Autodesk Inventor part; units mm, degrees
(part 2 of 4)
  circle A543 centre (81.83, 22.3) radius 1.125
  circle A544 centre (8.17, 19.76) radius 1.125
  circle A545 centre (10.71, 19.76) radius 1.125
  circle A546 centre (13.25, 19.76) radius 1.125
  circle A547 centre (15.79, 19.76) radius 1.125
  circle A548 centre (18.33, 19.76) radius 1.125
  circle A549 centre (20.87, 19.76) radius 1.125
  circle A550 centre (23.41, 19.76) radius 1.125
  circle A551 centre (25.95, 19.76) radius 1.125
  circle A552 centre (28.49, 19.76) radius 1.125
  circle A553 centre (31.03, 19.76) radius 1.125
  circle A554 centre (33.57, 19.76) radius 1.125
  circle A555 centre (36.11, 19.76) radius 1.125
  circle A556 centre (38.65, 19.76) radius 1.125
  circle A557 centre (41.19, 19.76) radius 1.125
  circle A558 centre (43.73, 19.76) radius 1.125
  circle A559 centre (46.27, 19.76) radius 1.125
  circle A560 centre (48.81, 19.76) radius 1.125
  circle A561 centre (51.35, 19.76) radius 1.125
  circle A562 centre (53.89, 19.76) radius 1.125
  circle A563 centre (56.43, 19.76) radius 1.125
  circle A564 centre (58.97, 19.76) radius 1.125
  circle A565 centre (61.51, 19.76) radius 1.125
  circle A566 centre (64.05, 19.76) radius 1.125
  circle A567 centre (66.59, 19.76) radius 1.125
  circle A568 centre (69.13, 19.76) radius 1.125
  circle A569 centre (71.67, 19.76) radius 1.125
  circle A570 centre (74.21, 19.76) radius 1.125
  circle A571 centre (76.75, 19.76) radius 1.125
  circle A572 centre (79.29, 19.76) radius 1.125
  circle A573 centre (81.83, 19.76) radius 1.125
  circle A574 centre (8.17, 17.22) radius 1.125
  circle A575 centre (10.71, 17.22) radius 1.125
  circle A576 centre (13.25, 17.22) radius 1.125
  circle A577 centre (15.79, 17.22) radius 1.125
  circle A578 centre (18.33, 17.22) radius 1.125
  circle A579 centre (20.87, 17.22) radius 1.125
  circle A580 centre (23.41, 17.22) radius 1.125
  circle A581 centre (25.95, 17.22) radius 1.125
  circle A582 centre (28.49, 17.22) radius 1.125
  circle A583 centre (31.03, 17.22) radius 1.125
  circle A584 centre (33.57, 17.22) radius 1.125
  circle A585 centre (36.11, 17.22) radius 1.125
  circle A586 centre (38.65, 17.22) radius 1.125
  circle A587 centre (41.19, 17.22) radius 1.125
  circle A588 centre (43.73, 17.22) radius 1.125
  circle A589 centre (46.27, 17.22) radius 1.125
  circle A590 centre (48.81, 17.22) radius 1.125
  circle A591 centre (51.35, 17.22) radius 1.125
  circle A592 centre (53.89, 17.22) radius 1.125
  circle A593 centre (56.43, 17.22) radius 1.125
  circle A594 centre (58.97, 17.22) radius 1.125
  circle A595 centre (61.51, 17.22) radius 1.125
  circle A596 centre (64.05, 17.22) radius 1.125
  circle A597 centre (66.59, 17.22) radius 1.125
  circle A598 centre (69.13, 17.22) radius 1.125
  circle A599 centre (71.67, 17.22) radius 1.125
  circle A600 centre (74.21, 17.22) radius 1.125
  circle A601 centre (76.75, 17.22) radius 1.125
  circle A602 centre (79.29, 17.22) radius 1.125
  circle A603 centre (81.83, 17.22) radius 1.125
  circle A604 centre (8.17, 14.68) radius 1.125
  circle A605 centre (10.71, 14.68) radius 1.125
  circle A606 centre (13.25, 14.68) radius 1.125
  circle A607 centre (15.79, 14.68) radius 1.125
  circle A608 centre (18.33, 14.68) radius 1.125
  circle A609 centre (20.87, 14.68) radius 1.125
  circle A610 centre (23.41, 14.68) radius 1.125
  circle A611 centre (25.95, 14.68) radius 1.125
  circle A612 centre (28.49, 14.68) radius 1.125
  circle A613 centre (31.03, 14.68) radius 1.125
  circle A614 centre (33.57, 14.68) radius 1.125
  circle A615 centre (36.11, 14.68) radius 1.125
  circle A616 centre (38.65, 14.68) radius 1.125
  circle A617 centre (41.19, 14.68) radius 1.125
  circle A618 centre (43.73, 14.68) radius 1.125
  circle A619 centre (46.27, 14.68) radius 1.125
  circle A620 centre (48.81, 14.68) radius 1.125
  circle A621 centre (51.35, 14.68) radius 1.125
  circle A622 centre (53.89, 14.68) radius 1.125
  circle A623 centre (56.43, 14.68) radius 1.125
  circle A624 centre (58.97, 14.68) radius 1.125
  circle A625 centre (61.51, 14.68) radius 1.125
  circle A626 centre (64.05, 14.68) radius 1.125
  circle A627 centre (66.59, 14.68) radius 1.125
  circle A628 centre (69.13, 14.68) radius 1.125
  circle A629 centre (71.67, 14.68) radius 1.125
  circle A630 centre (74.21, 14.68) radius 1.125
  circle A631 centre (76.75, 14.68) radius 1.125
  circle A632 centre (79.29, 14.68) radius 1.125
  circle A633 centre (81.83, 14.68) radius 1.125
  circle A634 centre (8.17, 12.14) radius 1.125
  circle A635 centre (10.71, 12.14) radius 1.125
  circle A636 centre (13.25, 12.14) radius 1.125
  circle A637 centre (15.79, 12.14) radius 1.125
  circle A638 centre (18.33, 12.14) radius 1.125
  circle A639 centre (20.87, 12.14) radius 1.125
  circle A640 centre (23.41, 12.14) radius 1.125
  circle A641 centre (25.95, 12.14) radius 1.125
  circle A642 centre (28.49, 12.14) radius 1.125
  circle A643 centre (31.03, 12.14) radius 1.125
  circle A644 centre (33.57, 12.14) radius 1.125
  circle A645 centre (36.11, 12.14) radius 1.125
  circle A646 centre (38.65, 12.14) radius 1.125
  circle A647 centre (41.19, 12.14) radius 1.125
  circle A648 centre (43.73, 12.14) radius 1.125
  circle A649 centre (46.27, 12.14) radius 1.125
  circle A650 centre (48.81, 12.14) radius 1.125
  circle A651 centre (51.35, 12.14) radius 1.125
  circle A652 centre (53.89, 12.14) radius 1.125
  circle A653 centre (56.43, 12.14) radius 1.125
  circle A654 centre (58.97, 12.14) radius 1.125
  circle A655 centre (61.51, 12.14) radius 1.125
  circle A656 centre (64.05, 12.14) radius 1.125
  circle A657 centre (66.59, 12.14) radius 1.125
  circle A658 centre (69.13, 12.14) radius 1.125
  circle A659 centre (71.67, 12.14) radius 1.125
  circle A660 centre (74.21, 12.14) radius 1.125
  circle A661 centre (76.75, 12.14) radius 1.125
  circle A662 centre (79.29, 12.14) radius 1.125
  circle A663 centre (81.83, 12.14) radius 1.125
  circle A664 centre (8.17, 9.6) radius 1.125
  circle A665 centre (10.71, 9.6) radius 1.125
  circle A666 centre (13.25, 9.6) radius 1.125
  circle A667 centre (15.79, 9.6) radius 1.125
  circle A668 centre (18.33, 9.6) radius 1.125
  circle A669 centre (20.87, 9.6) radius 1.125
  circle A670 centre (23.41, 9.6) radius 1.125
  circle A671 centre (25.95, 9.6) radius 1.125
  circle A672 centre (28.49, 9.6) radius 1.125
  circle A673 centre (31.03, 9.6) radius 1.125
  circle A674 centre (33.57, 9.6) radius 1.125
  circle A675 centre (36.11, 9.6) radius 1.125
  circle A676 centre (38.65, 9.6) radius 1.125
  circle A677 centre (41.19, 9.6) radius 1.125
  circle A678 centre (43.73, 9.6) radius 1.125
  circle A679 centre (46.27, 9.6) radius 1.125
  circle A680 centre (48.81, 9.6) radius 1.125
  circle A681 centre (51.35, 9.6) radius 1.125
  circle A682 centre (53.89, 9.6) radius 1.125
  circle A683 centre (56.43, 9.6) radius 1.125
  circle A684 centre (58.97, 9.6) radius 1.125
  circle A685 centre (61.51, 9.6) radius 1.125
  circle A686 centre (64.05, 9.6) radius 1.125
  circle A687 centre (66.59, 9.6) radius 1.125
  circle A688 centre (69.13, 9.6) radius 1.125
  circle A689 centre (71.67, 9.6) radius 1.125
  circle A690 centre (74.21, 9.6) radius 1.125
  circle A691 centre (76.75, 9.6) radius 1.125
  circle A692 centre (79.29, 9.6) radius 1.125
  circle A693 centre (81.83, 9.6) radius 1.125
  circle A694 centre (8.17, 7.06) radius 1.125
  circle A695 centre (10.71, 7.06) radius 1.125
  circle A696 centre (13.25, 7.06) radius 1.125
  circle A697 centre (15.79, 7.06) radius 1.125
  circle A698 centre (18.33, 7.06) radius 1.125
  circle A699 centre (20.87, 7.06) radius 1.125
  circle A700 centre (23.41, 7.06) radius 1.125
  circle A701 centre (25.95, 7.06) radius 1.125
  circle A702 centre (28.49, 7.06) radius 1.125
  circle A703 centre (31.03, 7.06) radius 1.125
  circle A704 centre (33.57, 7.06) radius 1.125
  circle A705 centre (36.11, 7.06) radius 1.125
  circle A706 centre (38.65, 7.06) radius 1.125
  circle A707 centre (41.19, 7.06) radius 1.125
  circle A708 centre (43.73, 7.06) radius 1.125
  circle A709 centre (46.27, 7.06) radius 1.125
  circle A710 centre (48.81, 7.06) radius 1.125
  circle A711 centre (51.35, 7.06) radius 1.125
  circle A712 centre (53.89, 7.06) radius 1.125
  circle A713 centre (56.43, 7.06) radius 1.125
  circle A714 centre (58.97, 7.06) radius 1.125
  circle A715 centre (61.51, 7.06) radius 1.125
  circle A716 centre (64.05, 7.06) radius 1.125
  circle A717 centre (66.59, 7.06) radius 1.125
  circle A718 centre (69.13, 7.06) radius 1.125
  circle A719 centre (71.67, 7.06) radius 1.125
  circle A720 centre (74.21, 7.06) radius 1.125
  circle A721 centre (76.75, 7.06) radius 1.125
  circle A722 centre (79.29, 7.06) radius 1.125
  circle A723 centre (81.83, 7.06) radius 1.125
  circle A724 centre (8.17, 4.52) radius 1.125
  circle A725 centre (10.71, 4.52) radius 1.125
  circle A726 centre (13.25, 4.52) radius 1.125
  circle A727 centre (15.79, 4.52) radius 1.125
  circle A728 centre (18.33, 4.52) radius 1.125
  circle A729 centre (20.87, 4.52) radius 1.125
  circle A730 centre (23.41, 4.52) radius 1.125
  circle A731 centre (25.95, 4.52) radius 1.125
  circle A732 centre (28.49, 4.52) radius 1.125
  circle A733 centre (31.03, 4.52) radius 1.125
  circle A734 centre (33.57, 4.52) radius 1.125
  circle A735 centre (36.11, 4.52) radius 1.125
  circle A736 centre (38.65, 4.52) radius 1.125
  circle A737 centre (41.19, 4.52) radius 1.125
  circle A738 centre (43.73, 4.52) radius 1.125
  circle A739 centre (46.27, 4.52) radius 1.125
  circle A740 centre (48.81, 4.52) radius 1.125
  circle A741 centre (51.35, 4.52) radius 1.125
  circle A742 centre (53.89, 4.52) radius 1.125
  circle A743 centre (56.43, 4.52) radius 1.125
  circle A744 centre (58.97, 4.52) radius 1.125
  circle A745 centre (61.51, 4.52) radius 1.125
  circle A746 centre (64.05, 4.52) radius 1.125
  circle A747 centre (66.59, 4.52) radius 1.125
  circle A748 centre (69.13, 4.52) radius 1.125
  circle A749 centre (71.67, 4.52) radius 1.125
  circle A750 centre (74.21, 4.52) radius 1.125
  circle A751 centre (76.75, 4.52) radius 1.125
  circle A752 centre (79.29, 4.52) radius 1.125
  circle A753 centre (81.83, 4.52) radius 1.125
  line L4 (0, 70) -> (0, 0) construction
  line L5 (0, 35) -> (90, 35) construction
  line L6 (45, 70) -> (45, 0) construction
  line L7 (0, 0) -> (90, 0) construction
  line L8 (43.73, 65.48) -> (46.27, 65.48) construction
  point P0 (45, 65.48)
  dimension "d9" = 2.25
  dimension "d12" = 2.54
  dimension "d15" = 2.54
  constraints: 750 centre point, 6 end point, 5 midpoint, 2 horizontal, 2 point on line, 1 vertical, 1498 other
  measures "d9" diameter of A0
  measures "d12" distance of A0.centre A5.centre
  measures "d15" distance of A0.centre A34.centre
extrude "PCB_Pads" add sketch "Sketch3" along normal blind 0.05
sketch "Sketch6" plane through (0, 0, 0) normal (0, -1, 0) x (1, 0, 0)
  arc A0 (2.6, -13.65) -> (2.6, -16.35) centre (2.6, -15) ccw construction
  line L0 (2.6, -16.35) -> (4.9, -16.35) construction
  arc A1 (4.9, -16.35) -> (4.9, -13.65) centre (4.9, -15) ccw construction
  line L1 (4.9, -13.65) -> (2.6, -13.65) construction
  arc A2 (2.6, -21.65) -> (2.6, -24.35) centre (2.6, -23) ccw construction
  line L2 (2.6, -24.35) -> (4.9, -24.35) construction
  arc A3 (4.9, -24.35) -> (4.9, -21.65) centre (4.9, -23) ccw construction
  line L3 (4.9, -21.65) -> (2.6, -21.65) construction
  arc A4 (2.6, -49.65) -> (2.6, -52.35) centre (2.6, -51) ccw construction
  line L4 (2.6, -52.35) -> (4.9, -52.35) construction
  arc A5 (4.9, -52.35) -> (4.9, -49.65) centre (4.9, -51) ccw construction
  line L5 (4.9, -49.65) -> (2.6, -49.65) construction
  arc A6 (2.6, -37.65) -> (2.6, -40.35) centre (2.6, -39) ccw construction
  line L6 (2.6, -40.35) -> (4.9, -40.35) construction
  arc A7 (4.9, -40.35) -> (4.9, -37.65) centre (4.9, -39) ccw construction
  line L7 (4.9, -37.65) -> (2.6, -37.65) construction
  arc A8 (2.6, -57.65) -> (2.6, -60.35) centre (2.6, -59) ccw construction
  line L8 (2.6, -60.35) -> (4.9, -60.35) construction
  arc A9 (4.9, -60.35) -> (4.9, -57.65) centre (4.9, -59) ccw construction
  line L9 (4.9, -57.65) -> (2.6, -57.65) construction
  arc A10 (2.6, -41.65) -> (2.6, -44.35) centre (2.6, -43) ccw construction
  line L10 (2.6, -44.35) -> (4.9, -44.35) construction
  arc A11 (4.9, -44.35) -> (4.9, -41.65) centre (4.9, -43) ccw construction
  line L11 (4.9, -41.65) -> (2.6, -41.65) construction
  arc A12 (85.1, -9.65) -> (85.1, -12.35) centre (85.1, -11) ccw construction
  line L12 (85.1, -12.35) -> (87.4, -12.35) construction
  arc A13 (87.4, -12.35) -> (87.4, -9.65) centre (87.4, -11) ccw construction
  line L13 (87.4, -9.65) -> (85.1, -9.65) construction
  arc A14 (85.1, -17.65) -> (85.1, -20.35) centre (85.1, -19) ccw construction
  line L14 (85.1, -20.35) -> (87.4, -20.35) construction
  arc A15 (87.4, -20.35) -> (87.4, -17.65) centre (87.4, -19) ccw construction
  line L15 (87.4, -17.65) -> (85.1, -17.65) construction
  arc A16 (85.1, -25.65) -> (85.1, -28.35) centre (85.1, -27) ccw construction
  line L16 (85.1, -28.35) -> (87.4, -28.35) construction
  arc A17 (87.4, -28.35) -> (87.4, -25.65) centre (87.4, -27) ccw construction
  line L17 (87.4, -25.65) -> (85.1, -25.65) construction
  arc A18 (85.1, -57.65) -> (85.1, -60.35) centre (85.1, -59) ccw construction
  line L18 (85.1, -60.35) -> (87.4, -60.35) construction
  arc A19 (87.4, -60.35) -> (87.4, -57.65) centre (87.4, -59) ccw construction
  line L19 (87.4, -57.65) -> (85.1, -57.65) construction
  arc A20 (85.1, -49.65) -> (85.1, -52.35) centre (85.1, -51) ccw construction
  line L20 (85.1, -52.35) -> (87.4, -52.35) construction
  arc A21 (87.4, -52.35) -> (87.4, -49.65) centre (87.4, -51) ccw construction
  line L21 (87.4, -49.65) -> (85.1, -49.65) construction
  arc A22 (85.1, -41.65) -> (85.1, -44.35) centre (85.1, -43) ccw construction
  line L22 (85.1, -44.35) -> (87.4, -44.35) construction
  arc A23 (87.4, -44.35) -> (87.4, -41.65) centre (87.4, -43) ccw construction
  line L23 (87.4, -41.65) -> (85.1, -41.65) construction
  arc A24 (87.4, -36.35) -> (87.4, -33.65) centre (87.4, -35) ccw construction
  line L24 (87.4, -33.65) -> (85.1, -33.65) construction
  arc A25 (85.1, -33.65) -> (85.1, -36.35) centre (85.1, -35) ccw construction
  line L25 (85.1, -36.35) -> (87.4, -36.35) construction
  arc A26 (85.1, -37.65) -> (85.1, -40.35) centre (85.1, -39) ccw construction
  line L26 (85.1, -40.35) -> (87.4, -40.35) construction
  arc A27 (87.4, -40.35) -> (87.4, -37.65) centre (87.4, -39) ccw construction
  line L27 (87.4, -37.65) -> (85.1, -37.65) construction
  arc A28 (85.1, -45.65) -> (85.1, -48.35) centre (85.1, -47) ccw construction
  line L28 (85.1, -48.35) -> (87.4, -48.35) construction
  arc A29 (87.4, -48.35) -> (87.4, -45.65) centre (87.4, -47) ccw construction
  line L29 (87.4, -45.65) -> (85.1, -45.65) construction
  arc A30 (85.1, -53.65) -> (85.1, -56.35) centre (85.1, -55) ccw construction
  line L30 (85.1, -56.35) -> (87.4, -56.35) construction
  arc A31 (87.4, -56.35) -> (87.4, -53.65) centre (87.4, -55) ccw construction
  line L31 (87.4, -53.65) -> (85.1, -53.65) construction
  arc A32 (85.1, -29.65) -> (85.1, -32.35) centre (85.1, -31) ccw construction
  line L32 (85.1, -32.35) -> (87.4, -32.35) construction
  arc A33 (87.4, -32.35) -> (87.4, -29.65) centre (87.4, -31) ccw construction
  line L33 (87.4, -29.65) -> (85.1, -29.65) construction
  arc A34 (85.1, -21.65) -> (85.1, -24.35) centre (85.1, -23) ccw construction
  line L34 (85.1, -24.35) -> (87.4, -24.35) construction
  arc A35 (87.4, -24.35) -> (87.4, -21.65) centre (87.4, -23) ccw construction
  line L35 (87.4, -21.65) -> (85.1, -21.65) construction
  arc A36 (85.1, -13.65) -> (85.1, -16.35) centre (85.1, -15) ccw construction
  line L36 (85.1, -16.35) -> (87.4, -16.35) construction
  arc A37 (87.4, -16.35) -> (87.4, -13.65) centre (87.4, -15) ccw construction
  line L37 (87.4, -13.65) -> (85.1, -13.65) construction
  arc A38 (4.9, -36.35) -> (4.9, -33.65) centre (4.9, -35) ccw construction
  line L38 (4.9, -33.65) -> (2.6, -33.65) construction
  arc A39 (2.6, -33.65) -> (2.6, -36.35) centre (2.6, -35) ccw construction
  line L39 (2.6, -36.35) -> (4.9, -36.35) construction
  arc A40 (2.6, -53.65) -> (2.6, -56.35) centre (2.6, -55) ccw construction
  line L40 (2.6, -56.35) -> (4.9, -56.35) construction
  arc A41 (4.9, -56.35) -> (4.9, -53.65) centre (4.9, -55) ccw construction
  line L41 (4.9, -53.65) -> (2.6, -53.65) construction
  arc A42 (2.6, -29.65) -> (2.6, -32.35) centre (2.6, -31) ccw construction
  line L42 (2.6, -32.35) -> (4.9, -32.35) construction
  arc A43 (4.9, -32.35) -> (4.9, -29.65) centre (4.9, -31) ccw construction
  line L43 (4.9, -29.65) -> (2.6, -29.65) construction
  arc A44 (2.6, -45.65) -> (2.6, -48.35) centre (2.6, -47) ccw construction
  line L44 (2.6, -48.35) -> (4.9, -48.35) construction
  arc A45 (4.9, -48.35) -> (4.9, -45.65) centre (4.9, -47) ccw construction
  line L45 (4.9, -45.65) -> (2.6, -45.65) construction
  arc A46 (2.6, -25.65) -> (2.6, -28.35) centre (2.6, -27) ccw construction
  line L46 (2.6, -28.35) -> (4.9, -28.35) construction
  arc A47 (4.9, -28.35) -> (4.9, -25.65) centre (4.9, -27) ccw construction
  line L47 (4.9, -25.65) -> (2.6, -25.65) construction
  arc A48 (4.9, -20.35) -> (4.9, -17.65) centre (4.9, -19) ccw construction
  line L48 (4.9, -17.65) -> (2.6, -17.65) construction
  arc A49 (2.6, -17.65) -> (2.6, -20.35) centre (2.6, -19) ccw construction
  line L49 (2.6, -20.35) -> (4.9, -20.35) construction
  arc A50 (2.6, -9.65) -> (2.6, -12.35) centre (2.6, -11) ccw construction
  line L50 (2.6, -12.35) -> (4.9, -12.35) construction
  arc A51 (4.9, -12.35) -> (4.9, -9.65) centre (4.9, -11) ccw construction
  line L51 (4.9, -9.65) -> (2.6, -9.65) construction
  circle A52 centre (79.29, -4.52) radius 1.125 construction
  circle A53 centre (74.21, -4.52) radius 1.125 construction
  circle A54 centre (69.13, -4.52) radius 1.125 construction
  circle A55 centre (64.05, -4.52) radius 1.125 construction
  circle A56 centre (58.97, -4.52) radius 1.125 construction
  circle A57 centre (53.89, -4.52) radius 1.125 construction
  circle A58 centre (48.81, -4.52) radius 1.125 construction
  circle A59 centre (43.73, -4.52) radius 1.125 construction
  circle A60 centre (38.65, -4.52) radius 1.125 construction
  circle A61 centre (33.57, -4.52) radius 1.125 construction
  circle A62 centre (28.49, -4.52) radius 1.125 construction
  circle A63 centre (23.41, -4.52) radius 1.125 construction
  circle A64 centre (18.33, -4.52) radius 1.125 construction
  circle A65 centre (13.25, -4.52) radius 1.125 construction
  circle A66 centre (8.17, -4.52) radius 1.125 construction
  circle A67 centre (79.29, -7.06) radius 1.125 construction
  circle A68 centre (74.21, -7.06) radius 1.125 construction
  circle A69 centre (69.13, -7.06) radius 1.125 construction
  circle A70 centre (64.05, -7.06) radius 1.125 construction
  circle A71 centre (58.97, -7.06) radius 1.125 construction
  circle A72 centre (53.89, -7.06) radius 1.125 construction
  circle A73 centre (48.81, -7.06) radius 1.125 construction
  circle A74 centre (43.73, -7.06) radius 1.125 construction
  circle A75 centre (38.65, -7.06) radius 1.125 construction
  circle A76 centre (33.57, -7.06) radius 1.125 construction
  circle A77 centre (28.49, -7.06) radius 1.125 construction
  circle A78 centre (23.41, -7.06) radius 1.125 construction
  circle A79 centre (18.33, -7.06) radius 1.125 construction
  circle A80 centre (13.25, -7.06) radius 1.125 construction
  circle A81 centre (8.17, -7.06) radius 1.125 construction
  circle A82 centre (79.29, -9.6) radius 1.125 construction
  circle A83 centre (74.21, -9.6) radius 1.125 construction
  circle A84 centre (69.13, -9.6) radius 1.125 construction
  circle A85 centre (64.05, -9.6) radius 1.125 construction
  circle A86 centre (58.97, -9.6) radius 1.125 construction
  circle A87 centre (53.89, -9.6) radius 1.125 construction
  circle A88 centre (48.81, -9.6) radius 1.125 construction
  circle A89 centre (43.73, -9.6) radius 1.125 construction
  circle A90 centre (38.65, -9.6) radius 1.125 construction
  circle A91 centre (33.57, -9.6) radius 1.125 construction
  circle A92 centre (28.49, -9.6) radius 1.125 construction
  circle A93 centre (23.41, -9.6) radius 1.125 construction
  circle A94 centre (18.33, -9.6) radius 1.125 construction
  circle A95 centre (13.25, -9.6) radius 1.125 construction
  circle A96 centre (8.17, -9.6) radius 1.125 construction
  circle A97 centre (79.29, -12.14) radius 1.125 construction
  circle A98 centre (74.21, -12.14) radius 1.125 construction
  circle A99 centre (69.13, -12.14) radius 1.125 construction
  circle A100 centre (64.05, -12.14) radius 1.125 construction
  circle A101 centre (58.97, -12.14) radius 1.125 construction
  circle A102 centre (53.89, -12.14) radius 1.125 construction
  circle A103 centre (48.81, -12.14) radius 1.125 construction
  circle A104 centre (43.73, -12.14) radius 1.125 construction
  circle A105 centre (38.65, -12.14) radius 1.125 construction
  circle A106 centre (33.57, -12.14) radius 1.125 construction
  circle A107 centre (28.49, -12.14) radius 1.125 construction
  circle A108 centre (23.41, -12.14) radius 1.125 construction
  circle A109 centre (18.33, -12.14) radius 1.125 construction
  circle A110 centre (13.25, -12.14) radius 1.125 construction
  circle A111 centre (8.17, -12.14) radius 1.125 construction
  circle A112 centre (79.29, -14.68) radius 1.125 construction
  circle A113 centre (74.21, -14.68) radius 1.125 construction
  circle A114 centre (69.13, -14.68) radius 1.125 construction
  circle A115 centre (64.05, -14.68) radius 1.125 construction
  circle A116 centre (58.97, -14.68) radius 1.125 construction
  circle A117 centre (53.89, -14.68) radius 1.125 construction
  circle A118 centre (48.81, -14.68) radius 1.125 construction
  circle A119 centre (43.73, -14.68) radius 1.125 construction
  circle A120 centre (38.65, -14.68) radius 1.125 construction
  circle A121 centre (33.57, -14.68) radius 1.125 construction
  circle A122 centre (28.49, -14.68) radius 1.125 construction
  circle A123 centre (23.41, -14.68) radius 1.125 construction
  circle A124 centre (18.33, -14.68) radius 1.125 construction
  circle A125 centre (13.25, -14.68) radius 1.125 construction
  circle A126 centre (8.17, -14.68) radius 1.125 construction
  circle A127 centre (79.29, -17.22) radius 1.125 construction
  circle A128 centre (74.21, -17.22) radius 1.125 construction
  circle A129 centre (69.13, -17.22) radius 1.125 construction
  circle A130 centre (64.05, -17.22) radius 1.125 construction
  circle A131 centre (58.97, -17.22) radius 1.125 construction
  circle A132 centre (53.89, -17.22) radius 1.125 construction
  circle A133 centre (48.81, -17.22) radius 1.125 construction
  circle A134 centre (43.73, -17.22) radius 1.125 construction
  circle A135 centre (38.65, -17.22) radius 1.125 construction
  circle A136 centre (33.57, -17.22) radius 1.125 construction
  circle A137 centre (28.49, -17.22) radius 1.125 construction
  circle A138 centre (23.41, -17.22) radius 1.125 construction
  circle A139 centre (18.33, -17.22) radius 1.125 construction
  circle A140 centre (13.25, -17.22) radius 1.125 construction
  circle A141 centre (8.17, -17.22) radius 1.125 construction
  circle A142 centre (79.29, -19.76) radius 1.125 construction
  circle A143 centre (74.21, -19.76) radius 1.125 construction
  circle A144 centre (69.13, -19.76) radius 1.125 construction
  circle A145 centre (64.05, -19.76) radius 1.125 construction
  circle A146 centre (58.97, -19.76) radius 1.125 construction
  circle A147 centre (53.89, -19.76) radius 1.125 construction
  circle A148 centre (48.81, -19.76) radius 1.125 construction
  circle A149 centre (43.73, -19.76) radius 1.125 construction
  circle A150 centre (38.65, -19.76) radius 1.125 construction
  circle A151 centre (33.57, -19.76) radius 1.125 construction
  circle A152 centre (28.49, -19.76) radius 1.125 construction
  circle A153 centre (23.41, -19.76) radius 1.125 construction
  circle A154 centre (18.33, -19.76) radius 1.125 construction
  circle A155 centre (13.25, -19.76) radius 1.125 construction
  circle A156 centre (8.17, -19.76) radius 1.125 construction
  circle A157 centre (79.29, -22.3) radius 1.125 construction
  circle A158 centre (74.21, -22.3) radius 1.125 construction
  circle A159 centre (69.13, -22.3) radius 1.125 construction
  circle A160 centre (64.05, -22.3) radius 1.125 construction
  circle A161 centre (58.97, -22.3) radius 1.125 construction
  circle A162 centre (53.89, -22.3) radius 1.125 construction
  circle A163 centre (48.81, -22.3) radius 1.125 construction
  circle A164 centre (43.73, -22.3) radius 1.125 construction
  circle A165 centre (38.65, -22.3) radius 1.125 construction
  circle A166 centre (33.57, -22.3) radius 1.125 construction
  circle A167 centre (28.49, -22.3) radius 1.125 construction
  circle A168 centre (23.41, -22.3) radius 1.125 construction
  circle A169 centre (18.33, -22.3) radius 1.125 construction
  circle A170 centre (13.25, -22.3) radius 1.125 construction
  circle A171 centre (8.17, -22.3) radius 1.125 construction
  circle A172 centre (79.29, -24.84) radius 1.125 construction
  circle A173 centre (74.21, -24.84) radius 1.125 construction
  circle A174 centre (69.13, -24.84) radius 1.125 construction
  circle A175 centre (64.05, -24.84) radius 1.125 construction
  circle A176 centre (58.97, -24.84) radius 1.125 construction
  circle A177 centre (53.89, -24.84) radius 1.125 construction
  circle A178 centre (48.81, -24.84) radius 1.125 construction
  circle A179 centre (43.73, -24.84) radius 1.125 construction
  circle A180 centre (38.65, -24.84) radius 1.125 construction
  circle A181 centre (33.57, -24.84) radius 1.125 construction
  circle A182 centre (28.49, -24.84) radius 1.125 construction
  circle A183 centre (23.41, -24.84) radius 1.125 construction
  circle A184 centre (18.33, -24.84) radius 1.125 construction
  circle A185 centre (13.25, -24.84) radius 1.125 construction
  circle A186 centre (8.17, -24.84) radius 1.125 construction
  circle A187 centre (79.29, -27.38) radius 1.125 construction
  circle A188 centre (74.21, -27.38) radius 1.125 construction
  circle A189 centre (69.13, -27.38) radius 1.125 construction
  circle A190 centre (64.05, -27.38) radius 1.125 construction
  circle A191 centre (58.97, -27.38) radius 1.125 construction
  circle A192 centre (53.89, -27.38) radius 1.125 construction
  circle A193 centre (48.81, -27.38) radius 1.125 construction
  circle A194 centre (43.73, -27.38) radius 1.125 construction
  circle A195 centre (38.65, -27.38) radius 1.125 construction
  circle A196 centre (33.57, -27.38) radius 1.125 construction
  circle A197 centre (28.49, -27.38) radius 1.125 construction
  circle A198 centre (23.41, -27.38) radius 1.125 construction
  circle A199 centre (18.33, -27.38) radius 1.125 construction
  circle A200 centre (13.25, -27.38) radius 1.125 construction
  circle A201 centre (8.17, -27.38) radius 1.125 construction
  circle A202 centre (79.29, -29.92) radius 1.125 construction
  circle A203 centre (74.21, -29.92) radius 1.125 construction
  circle A204 centre (69.13, -29.92) radius 1.125 construction
  circle A205 centre (64.05, -29.92) radius 1.125 construction
  circle A206 centre (58.97, -29.92) radius 1.125 construction
  circle A207 centre (53.89, -29.92) radius 1.125 construction
  circle A208 centre (48.81, -29.92) radius 1.125 construction
  circle A209 centre (43.73, -29.92) radius 1.125 construction
  circle A210 centre (38.65, -29.92) radius 1.125 construction
  circle A211 centre (33.57, -29.92) radius 1.125 construction
  circle A212 centre (28.49, -29.92) radius 1.125 construction
  circle A213 centre (23.41, -29.92) radius 1.125 construction
  circle A214 centre (18.33, -29.92) radius 1.125 construction
  circle A215 centre (13.25, -29.92) radius 1.125 construction
  circle A216 centre (8.17, -29.92) radius 1.125 construction
  circle A217 centre (79.29, -32.46) radius 1.125 construction
  circle A218 centre (74.21, -32.46) radius 1.125 construction
  circle A219 centre (69.13, -32.46) radius 1.125 construction
  circle A220 centre (64.05, -32.46) radius 1.125 construction
  circle A221 centre (58.97, -32.46) radius 1.125 construction
  circle A222 centre (53.89, -32.46) radius 1.125 construction
  circle A223 centre (48.81, -32.46) radius 1.125 construction
  circle A224 centre (43.73, -32.46) radius 1.125 construction
  circle A225 centre (38.65, -32.46) radius 1.125 construction
  circle A226 centre (33.57, -32.46) radius 1.125 construction
  circle A227 centre (28.49, -32.46) radius 1.125 construction
  circle A228 centre (23.41, -32.46) radius 1.125 construction
  circle A229 centre (18.33, -32.46) radius 1.125 construction
  circle A230 centre (13.25, -32.46) radius 1.125 construction
  circle A231 centre (8.17, -32.46) radius 1.125 construction
  circle A232 centre (79.29, -35) radius 1.125 construction
  circle A233 centre (74.21, -35) radius 1.125 construction
  circle A234 centre (69.13, -35) radius 1.125 construction
  circle A235 centre (64.05, -35) radius 1.125 construction
  circle A236 centre (58.97, -35) radius 1.125 construction
  circle A237 centre (53.89, -35) radius 1.125 construction
  circle A238 centre (48.81, -35) radius 1.125 construction
  circle A239 centre (43.73, -35) radius 1.125 construction
  circle A240 centre (38.65, -35) radius 1.125 construction
  circle A241 centre (33.57, -35) radius 1.125 construction
  circle A242 centre (28.49, -35) radius 1.125 construction
  circle A243 centre (23.41, -35) radius 1.125 construction
  circle A244 centre (18.33, -35) radius 1.125 construction
  circle A245 centre (13.25, -35) radius 1.125 construction
  circle A246 centre (8.17, -35) radius 1.125 construction
  circle A247 centre (79.29, -37.54) radius 1.125 construction
  circle A248 centre (74.21, -37.54) radius 1.125 construction
  circle A249 centre (69.13, -37.54) radius 1.125 construction
  circle A250 centre (64.05, -37.54) radius 1.125 construction
  circle A251 centre (58.97, -37.54) radius 1.125 construction
  circle A252 centre (53.89, -37.54) radius 1.125 construction
  circle A253 centre (48.81, -37.54) radius 1.125 construction
  circle A254 centre (43.73, -37.54) radius 1.125 construction
  circle A255 centre (38.65, -37.54) radius 1.125 construction
  circle A256 centre (33.57, -37.54) radius 1.125 construction
  circle A257 centre (28.49, -37.54) radius 1.125 construction
  circle A258 centre (23.41, -37.54) radius 1.125 construction
  circle A259 centre (18.33, -37.54) radius 1.125 construction
  circle A260 centre (13.25, -37.54) radius 1.125 construction
  circle A261 centre (8.17, -37.54) radius 1.125 construction
  circle A262 centre (79.29, -40.08) radius 1.125 construction
  circle A263 centre (74.21, -40.08) radius 1.125 construction
  circle A264 centre (69.13, -40.08) radius 1.125 construction
  circle A265 centre (64.05, -40.08) radius 1.125 construction
  circle A266 centre (58.97, -40.08) radius 1.125 construction
  circle A267 centre (53.89, -40.08) radius 1.125 construction
  circle A268 centre (48.81, -40.08) radius 1.125 construction
  circle A269 centre (43.73, -40.08) radius 1.125 construction
  circle A270 centre (38.65, -40.08) radius 1.125 construction
  circle A271 centre (33.57, -40.08) radius 1.125 construction
  circle A272 centre (28.49, -40.08) radius 1.125 construction
  circle A273 centre (23.41, -40.08) radius 1.125 construction
  circle A274 centre (18.33, -40.08) radius 1.125 construction
  circle A275 centre (13.25, -40.08) radius 1.125 construction
  circle A276 centre (8.17, -40.08) radius 1.125 construction
  circle A277 centre (79.29, -42.62) radius 1.125 construction
  circle A278 centre (74.21, -42.62) radius 1.125 construction
  circle A279 centre (69.13, -42.62) radius 1.125 construction
  circle A280 centre (64.05, -42.62) radius 1.125 construction
  circle A281 centre (58.97, -42.62) radius 1.125 construction
  circle A282 centre (53.89, -42.62) radius 1.125 construction
  circle A283 centre (48.81, -42.62) radius 1.125 construction
  circle A284 centre (43.73, -42.62) radius 1.125 construction
  circle A285 centre (38.65, -42.62) radius 1.125 construction
  circle A286 centre (33.57, -42.62) radius 1.125 construction
  circle A287 centre (28.49, -42.62) radius 1.125 construction
  circle A288 centre (23.41, -42.62) radius 1.125 construction
  circle A289 centre (18.33, -42.62) radius 1.125 construction
  circle A290 centre (13.25, -42.62) radius 1.125 construction
  circle A291 centre (8.17, -42.62) radius 1.125 construction
  circle A292 centre (79.29, -45.16) radius 1.125 construction
  circle A293 centre (74.21, -45.16) radius 1.125 construction
  circle A294 centre (69.13, -45.16) radius 1.125 construction
  circle A295 centre (64.05, -45.16) radius 1.125 construction
  circle A296 centre (58.97, -45.16) radius 1.125 construction
  circle A297 centre (53.89, -45.16) radius 1.125 construction
  circle A298 centre (48.81, -45.16) radius 1.125 construction
  circle A299 centre (43.73, -45.16) radius 1.125 construction
  circle A300 centre (38.65, -45.16) radius 1.125 construction
  circle A301 centre (33.57, -45.16) radius 1.125 construction
  circle A302 centre (28.49, -45.16) radius 1.125 construction
  circle A303 centre (23.41, -45.16) radius 1.125 construction
  circle A304 centre (18.33, -45.16) radius 1.125 construction
  circle A305 centre (13.25, -45.16) radius 1.125 construction
  circle A306 centre (8.17, -45.16) radius 1.125 construction
  circle A307 centre (79.29, -47.7) radius 1.125 construction
  circle A308 centre (74.21, -47.7) radius 1.125 construction
  circle A309 centre (69.13, -47.7) radius 1.125 construction
  circle A310 centre (64.05, -47.7) radius 1.125 construction
  circle A311 centre (58.97, -47.7) radius 1.125 construction
  circle A312 centre (53.89, -47.7) radius 1.125 construction
  circle A313 centre (48.81, -47.7) radius 1.125 construction
  circle A314 centre (43.73, -47.7) radius 1.125 construction
  circle A315 centre (38.65, -47.7) radius 1.125 construction
  circle A316 centre (33.57, -47.7) radius 1.125 construction
  circle A317 centre (28.49, -47.7) radius 1.125 construction
  circle A318 centre (23.41, -47.7) radius 1.125 construction
  circle A319 centre (18.33, -47.7) radius 1.125 construction
  circle A320 centre (13.25, -47.7) radius 1.125 construction
  circle A321 centre (8.17, -47.7) radius 1.125 construction
  circle A322 centre (79.29, -50.24) radius 1.125 construction
  circle A323 centre (74.21, -50.24) radius 1.125 construction
  circle A324 centre (69.13, -50.24) radius 1.125 construction
  circle A325 centre (64.05, -50.24) radius 1.125 construction
  circle A326 centre (58.97, -50.24) radius 1.125 construction
  circle A327 centre (53.89, -50.24) radius 1.125 construction
  circle A328 centre (48.81, -50.24) radius 1.125 construction
  circle A329 centre (43.73, -50.24) radius 1.125 construction
  circle A330 centre (38.65, -50.24) radius 1.125 construction
  circle A331 centre (33.57, -50.24) radius 1.125 construction
  circle A332 centre (28.49, -50.24) radius 1.125 construction
  circle A333 centre (23.41, -50.24) radius 1.125 construction
  circle A334 centre (18.33, -50.24) radius 1.125 construction
  circle A335 centre (13.25, -50.24) radius 1.125 construction
  circle A336 centre (8.17, -50.24) radius 1.125 construction
  circle A337 centre (79.29, -52.78) radius 1.125 construction
  circle A338 centre (74.21, -52.78) radius 1.125 construction
  circle A339 centre (69.13, -52.78) radius 1.125 construction
  circle A340 centre (64.05, -52.78) radius 1.125 construction
  circle A341 centre (58.97, -52.78) radius 1.125 construction
  circle A342 centre (53.89, -52.78) radius 1.125 construction
  circle A343 centre (48.81, -52.78) radius 1.125 construction
  circle A344 centre (43.73, -52.78) radius 1.125 construction
  circle A345 centre (38.65, -52.78) radius 1.125 construction
  circle A346 centre (33.57, -52.78) radius 1.125 construction
  circle A347 centre (28.49, -52.78) radius 1.125 construction
  circle A348 centre (23.41, -52.78) radius 1.125 construction
  circle A349 centre (18.33, -52.78) radius 1.125 construction
  circle A350 centre (13.25, -52.78) radius 1.125 construction
  circle A351 centre (8.17, -52.78) radius 1.125 construction
  circle A352 centre (79.29, -55.32) radius 1.125 construction
  circle A353 centre (74.21, -55.32) radius 1.125 construction
  circle A354 centre (69.13, -55.32) radius 1.125 construction
  circle A355 centre (64.05, -55.32) radius 1.125 construction
  circle A356 centre (58.97, -55.32) radius 1.125 construction
  circle A357 centre (53.89, -55.32) radius 1.125 construction
  circle A358 centre (48.81, -55.32) radius 1.125 construction
  circle A359 centre (43.73, -55.32) radius 1.125 construction
  circle A360 centre (38.65, -55.32) radius 1.125 construction
  circle A361 centre (33.57, -55.32) radius 1.125 construction
  circle A362 centre (28.49, -55.32) radius 1.125 construction
  circle A363 centre (23.41, -55.32) radius 1.125 construction
  circle A364 centre (18.33, -55.32) radius 1.125 construction
  circle A365 centre (13.25, -55.32) radius 1.125 construction
  circle A366 centre (8.17, -55.32) radius 1.125 construction
  circle A367 centre (79.29, -57.86) radius 1.125 construction
  circle A368 centre (74.21, -57.86) radius 1.125 construction
  circle A369 centre (69.13, -57.86) radius 1.125 construction
  circle A370 centre (64.05, -57.86) radius 1.125 construction
  circle A371 centre (58.97, -57.86) radius 1.125 construction
  circle A372 centre (53.89, -57.86) radius 1.125 construction
  circle A373 centre (48.81, -57.86) radius 1.125 construction
  circle A374 centre (43.73, -57.86) radius 1.125 construction
  circle A375 centre (38.65, -57.86) radius 1.125 construction
  circle A376 centre (33.57, -57.86) radius 1.125 construction
  circle A377 centre (28.49, -57.86) radius 1.125 construction
  circle A378 centre (23.41, -57.86) radius 1.125 construction
  circle A379 centre (18.33, -57.86) radius 1.125 construction
  circle A380 centre (13.25, -57.86) radius 1.125 construction
  circle A381 centre (8.17, -57.86) radius 1.125 construction
  circle A382 centre (79.29, -60.4) radius 1.125 construction
  circle A383 centre (74.21, -60.4) radius 1.125 construction
  circle A384 centre (69.13, -60.4) radius 1.125 construction
  circle A385 centre (64.05, -60.4) radius 1.125 construction
  circle A386 centre (58.97, -60.4) radius 1.125 construction
  circle A387 centre (53.89, -60.4) radius 1.125 construction
  circle A388 centre (48.81, -60.4) radius 1.125 construction
  circle A389 centre (43.73, -60.4) radius 1.125 construction
  circle A390 centre (38.65, -60.4) radius 1.125 construction
  circle A391 centre (33.57, -60.4) radius 1.125 construction
  circle A392 centre (28.49, -60.4) radius 1.125 construction
  circle A393 centre (23.41, -60.4) radius 1.125 construction
  circle A394 centre (18.33, -60.4) radius 1.125 construction
  circle A395 centre (13.25, -60.4) radius 1.125 construction
  circle A396 centre (8.17, -60.4) radius 1.125 construction
  circle A397 centre (79.29, -62.94) radius 1.125 construction
  circle A398 centre (74.21, -62.94) radius 1.125 construction
  circle A399 centre (69.13, -62.94) radius 1.125 construction
  circle A400 centre (64.05, -62.94) radius 1.125 construction
  circle A401 centre (58.97, -62.94) radius 1.125 construction
  circle A402 centre (53.89, -62.94) radius 1.125 construction
  circle A403 centre (48.81, -62.94) radius 1.125 construction
  circle A404 centre (43.73, -62.94) radius 1.125 construction
  circle A405 centre (38.65, -62.94) radius 1.125 construction
  circle A406 centre (33.57, -62.94) radius 1.125 construction
  circle A407 centre (28.49, -62.94) radius 1.125 construction
  circle A408 centre (23.41, -62.94) radius 1.125 construction
  circle A409 centre (18.33, -62.94) radius 1.125 construction
  circle A410 centre (13.25, -62.94) radius 1.125 construction
  circle A411 centre (8.17, -62.94) radius 1.125 construction
  circle A412 centre (79.29, -65.48) radius 1.125 construction
  circle A413 centre (74.21, -65.48) radius 1.125 construction
  circle A414 centre (69.13, -65.48) radius 1.125 construction
  circle A415 centre (64.05, -65.48) radius 1.125 construction
  circle A416 centre (58.97, -65.48) radius 1.125 construction
  circle A417 centre (53.89, -65.48) radius 1.125 construction
  circle A418 centre (48.81, -65.48) radius 1.125 construction
  circle A419 centre (43.73, -65.48) radius 1.125 construction
  circle A420 centre (38.65, -65.48) radius 1.125 construction
  circle A421 centre (33.57, -65.48) radius 1.125 construction
  circle A422 centre (28.49, -65.48) radius 1.125 construction
  circle A423 centre (23.41, -65.48) radius 1.125 construction
  circle A424 centre (18.33, -65.48) radius 1.125 construction
  circle A425 centre (13.25, -65.48) radius 1.125 construction
  circle A426 centre (8.17, -65.48) radius 1.125 construction
  circle A427 centre (10.71, -65.48) radius 1.125 construction
  circle A428 centre (15.79, -65.48) radius 1.125 construction
  circle A429 centre (20.87, -65.48) radius 1.125 construction
  circle A430 centre (25.95, -65.48) radius 1.125 construction
  circle A431 centre (31.03, -65.48) radius 1.125 construction
  circle A432 centre (36.11, -65.48) radius 1.125 construction
  circle A433 centre (41.19, -65.48) radius 1.125 construction
  circle A434 centre (46.27, -65.48) radius 1.125 construction
  circle A435 centre (51.35, -65.48) radius 1.125 construction
  circle A436 centre (56.43, -65.48) radius 1.125 construction
  circle A437 centre (61.51, -65.48) radius 1.125 construction
  circle A438 centre (66.59, -65.48) radius 1.125 construction
  circle A439 centre (71.67, -65.48) radius 1.125 construction
  circle A440 centre (76.75, -65.48) radius 1.125 construction
  circle A441 centre (81.83, -65.48) radius 1.125 construction
  circle A442 centre (10.71, -62.94) radius 1.125 construction
  circle A443 centre (15.79, -62.94) radius 1.125 construction
  circle A444 centre (20.87, -62.94) radius 1.125 construction
  circle A445 centre (25.95, -62.94) radius 1.125 construction
  circle A446 centre (31.03, -62.94) radius 1.125 construction
  circle A447 centre (36.11, -62.94) radius 1.125 construction
  circle A448 centre (41.19, -62.94) radius 1.125 construction
  circle A449 centre (46.27, -62.94) radius 1.125 construction
  circle A450 centre (51.35, -62.94) radius 1.125 construction
  circle A451 centre (56.43, -62.94) radius 1.125 construction
  circle A452 centre (61.51, -62.94) radius 1.125 construction
  circle A453 centre (66.59, -62.94) radius 1.125 construction
  circle A454 centre (71.67, -62.94) radius 1.125 construction
  circle A455 centre (76.75, -62.94) radius 1.125 construction
  circle A456 centre (81.83, -62.94) radius 1.125 construction
  circle A457 centre (10.71, -60.4) radius 1.125 construction
  circle A458 centre (15.79, -60.4) radius 1.125 construction
  circle A459 centre (20.87, -60.4) radius 1.125 construction
  circle A460 centre (25.95, -60.4) radius 1.125 construction
  circle A461 centre (31.03, -60.4) radius 1.125 construction
  circle A462 centre (36.11, -60.4) radius 1.125 construction
  circle A463 centre (41.19, -60.4) radius 1.125 construction
  circle A464 centre (46.27, -60.4) radius 1.125 construction
  circle A465 centre (51.35, -60.4) radius 1.125 construction
  circle A466 centre (56.43, -60.4) radius 1.125 construction
  circle A467 centre (61.51, -60.4) radius 1.125 construction
  circle A468 centre (66.59, -60.4) radius 1.125 construction
  circle A469 centre (71.67, -60.4) radius 1.125 construction
  circle A470 centre (76.75, -60.4) radius 1.125 construction
  circle A471 centre (81.83, -60.4) radius 1.125 construction
  circle A472 centre (10.71, -57.86) radius 1.125 construction
  circle A473 centre (15.79, -57.86) radius 1.125 construction
  circle A474 centre (20.87, -57.86) radius 1.125 construction
  circle A475 centre (25.95, -57.86) radius 1.125 construction
  circle A476 centre (31.03, -57.86) radius 1.125 construction
  circle A477 centre (36.11, -57.86) radius 1.125 construction
  circle A478 centre (41.19, -57.86) radius 1.125 construction
  circle A479 centre (46.27, -57.86) radius 1.125 construction
  circle A480 centre (51.35, -57.86) radius 1.125 construction
  circle A481 centre (56.43, -57.86) radius 1.125 construction
  circle A482 centre (61.51, -57.86) radius 1.125 construction
  circle A483 centre (66.59, -57.86) radius 1.125 construction
  circle A484 centre (71.67, -57.86) radius 1.125 construction
  circle A485 centre (76.75, -57.86) radius 1.125 construction
  circle A486 centre (81.83, -57.86) radius 1.125 construction
  circle A487 centre (10.71, -55.32) radius 1.125 construction
  circle A488 centre (15.79, -55.32) radius 1.125 construction
  circle A489 centre (20.87, -55.32) radius 1.125 construction
  circle A490 centre (25.95, -55.32) radius 1.125 construction
  circle A491 centre (31.03, -55.32) radius 1.125 construction
  circle A492 centre (36.11, -55.32) radius 1.125 construction
  circle A493 centre (41.19, -55.32) radius 1.125 construction
  circle A494 centre (46.27, -55.32) radius 1.125 construction
  circle A495 centre (51.35, -55.32) radius 1.125 construction
  circle A496 centre (56.43, -55.32) radius 1.125 construction
  circle A497 centre (61.51, -55.32) radius 1.125 construction
  circle A498 centre (66.59, -55.32) radius 1.125 construction
  circle A499 centre (71.67, -55.32) radius 1.125 construction
  circle A500 centre (76.75, -55.32) radius 1.125 construction
  circle A501 centre (81.83, -55.32) radius 1.125 construction
  circle A502 centre (10.71, -52.78) radius 1.125 construction
  circle A503 centre (15.79, -52.78) radius 1.125 construction
  circle A504 centre (20.87, -52.78) radius 1.125 construction
  circle A505 centre (25.95, -52.78) radius 1.125 construction
  circle A506 centre (31.03, -52.78) radius 1.125 construction
  circle A507 centre (36.11, -52.78) radius 1.125 construction
  circle A508 centre (41.19, -52.78) radius 1.125 construction
  circle A509 centre (46.27, -52.78) radius 1.125 construction
  circle A510 centre (51.35, -52.78) radius 1.125 construction
  circle A511 centre (56.43, -52.78) radius 1.125 construction
  circle A512 centre (61.51, -52.78) radius 1.125 construction
  circle A513 centre (66.59, -52.78) radius 1.125 construction
  circle A514 centre (71.67, -52.78) radius 1.125 construction
  circle A515 centre (76.75, -52.78) radius 1.125 construction
  circle A516 centre (81.83, -52.78) radius 1.125 construction
  circle A517 centre (10.71, -50.24) radius 1.125 construction
  circle A518 centre (15.79, -50.24) radius 1.125 construction
  circle A519 centre (20.87, -50.24) radius 1.125 construction
  circle A520 centre (25.95, -50.24) radius 1.125 construction
  circle A521 centre (31.03, -50.24) radius 1.125 construction
  circle A522 centre (36.11, -50.24) radius 1.125 construction
  circle A523 centre (41.19, -50.24) radius 1.125 construction
  circle A524 centre (46.27, -50.24) radius 1.125 construction
  circle A525 centre (51.35, -50.24) radius 1.125 construction
  circle A526 centre (56.43, -50.24) radius 1.125 construction
  circle A527 centre (61.51, -50.24) radius 1.125 construction
  circle A528 centre (66.59, -50.24) radius 1.125 construction
  circle A529 centre (71.67, -50.24) radius 1.125 construction
  circle A530 centre (76.75, -50.24) radius 1.125 construction
  circle A531 centre (81.83, -50.24) radius 1.125 construction
  circle A532 centre (10.71, -47.7) radius 1.125 construction
  circle A533 centre (15.79, -47.7) radius 1.125 construction
  circle A534 centre (20.87, -47.7) radius 1.125 construction
  circle A535 centre (25.95, -47.7) radius 1.125 construction
  circle A536 centre (31.03, -47.7) radius 1.125 construction
  circle A537 centre (36.11, -47.7) radius 1.125 construction
  circle A538 centre (41.19, -47.7) radius 1.125 construction
  circle A539 centre (46.27, -47.7) radius 1.125 construction
  circle A540 centre (51.35, -47.7) radius 1.125 construction
  circle A541 centre (56.43, -47.7) radius 1.125 construction
  circle A542 centre (61.51, -47.7) radius 1.125 construction
  circle A543 centre (66.59, -47.7) radius 1.125 construction
  circle A544 centre (71.67, -47.7) radius 1.125 construction
  circle A545 centre (76.75, -47.7) radius 1.125 construction
  circle A546 centre (81.83, -47.7) radius 1.125 construction
  circle A547 centre (10.71, -45.16) radius 1.125 construction
  circle A548 centre (15.79, -45.16) radius 1.125 construction
  circle A549 centre (20.87, -45.16) radius 1.125 construction
  circle A550 centre (25.95, -45.16) radius 1.125 construction
  circle A551 centre (31.03, -45.16) radius 1.125 construction
  circle A552 centre (36.11, -45.16) radius 1.125 construction
  circle A553 centre (41.19, -45.16) radius 1.125 construction
  circle A554 centre (46.27, -45.16) radius 1.125 construction
  circle A555 centre (51.35, -45.16) radius 1.125 construction
  circle A556 centre (56.43, -45.16) radius 1.125 construction
  circle A557 centre (61.51, -45.16) radius 1.125 construction
  circle A558 centre (66.59, -45.16) radius 1.125 construction
  circle A559 centre (71.67, -45.16) radius 1.125 construction
  circle A560 centre (76.75, -45.16) radius 1.125 construction
  circle A561 centre (81.83, -45.16) radius 1.125 construction
  circle A562 centre (10.71, -42.62) radius 1.125 construction
  circle A563 centre (15.79, -42.62) radius 1.125 construction
  circle A564 centre (20.87, -42.62) radius 1.125 construction